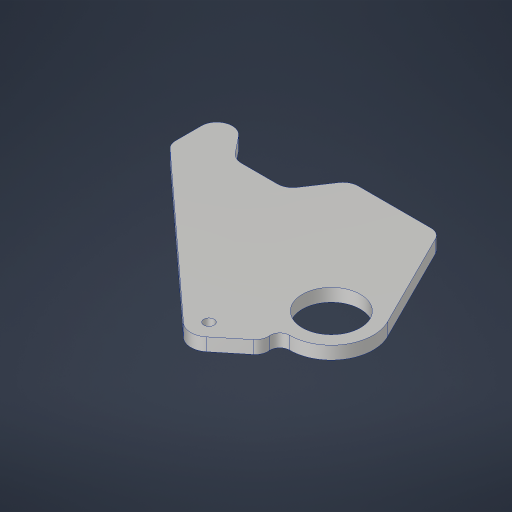
# Autodesk Inventor part: CL4-004
Saved by Autodesk Inventor 2023.4 (Build 274418000, 418)
## iProperties
Created: 2025-02-03
Part Number: CL4-004
Material: Aluminum 6061
Document SubType Name: Modeling
Designer: brand
Density: 2.7 g/cm^3
Appearance: Aluminum - Flat
Author: brand
Autodesk Inventor part; units mm, degrees
ref_plane "YZ Plane" through (0, 0, 0) normal (1, 0, 0) x (0, 1, 0)
ref_plane "XZ Plane" through (0, 0, 0) normal (0, 1, 0) x (-1, 0, 0)
ref_plane "XY Plane" through (0, 0, 0) normal (0, 0, 1) x (1, 0, 0)
sketch "Sketch1" plane through (0, 0, 0) normal (0, 1, 0) x (-1, 0, 0)
  circle A0 centre (76.2, -63.1164) radius 16.7005 construction
  line L0 (63.5, -40.9794) -> (88.9, -40.9794)
  line L1 (88.9, -40.9794) -> (101.6, -56.8544)
  line L2 (101.6, -56.8544) -> (111.125, -56.8544)
  line L3 (111.125, -56.8544) -> (111.125, -31.4544)
  line L4 (111.125, -31.4544) -> (31.4102, 41.4928)
  line L5 (63.5, -40.9794) -> (50.8, -60.0294)
  line L6 (50.8, -60.0294) -> (6.9413, -60.0294)
  circle A1 centre (0, 0) radius 14.2875
  circle A2 centre (0, 0) radius 20.6375 construction
  line L7 (6.9413, -60.0294) -> (-18.4587, -9.2294)
  circle A3 centre (0, 25.4) radius 4.7625 construction
  circle A4 centre (25.4, 34.925) radius 2.5527 construction
  circle A5 centre (25.4, 34.925) radius 8.9027 construction
  line L8 (19.7688, 41.8204) -> (3.5498, 28.575)
  arc A6 (0, 20.6375) -> (3.5498, 28.575) centre (0, 25.4) ccw
  arc A7 (0, 20.6375) -> (-18.4587, -9.2294) centre (0, 0) ccw
  arc A8 (31.4102, 41.4928) -> (19.7688, 41.8204) centre (25.4, 34.925) ccw
  point P0 (76.2, -40.9794)
  dimension "d0" = 33.401
  dimension "d1" = 28.575
  dimension "d2" = 6.35
  dimension "d3" = 9.525
  dimension "d4" = 25.4
  dimension "d5" = 5.1054
  dimension "d6" = 6.35
  dimension "d7" = 25.4
  dimension "d8" = 9.525
  dimension "d9" = 25.4
  dimension "d10" = 50.8
  dimension "d11" = 19.05
  dimension "d12" = 12.7
  dimension "d13" = 25.4
  dimension "d15" = 76.2
  dimension "d16" = 76.2
  dimension "d17" = 12.7
  dimension "d18" = 3.175
  dimension "d19" = 9.525
  dimension "d20" = 25.4
  dimension "d21" = 3.175
  dimension "d22" = 63.1164
  constraints: 18 end point, 10 point on circle, 8 centre point, 4 coincident, 2 horizontal, 2 tangent, 1 concentric, 1 midpoint, 1 parallel, 1 vertical, 1 vertical alignment, 4 other
  measures "d0" diameter of A0
  measures "d1" diameter of A1
  measures "d3" diameter of A3
  measures "d4" distance of A3.centre point (0, 0)
  measures "d5" diameter of A4
  measures "d6" radial gap between concentric circles of A4 A5
  measures "d7" horizontal distance of A4.centre A3.centre
  measures "d8" vertical distance of A3.centre A4.centre
  measures "d9" horizontal distance of L7.end L6.end
  measures "d10" vertical distance of L7.end L6.end
  measures "d11" vertical distance of L0.start L5.end
  measures "d12" horizontal distance of L0.start L5.end
  measures "d13" distance of L0.start L0.end
  measures "d15" horizontal distance of point (0, 0) point (76.2, -40.979)
  measures "d16" horizontal distance of point (0, 0) A0.centre
  measures "d17" horizontal distance of L0.end L1.end
  measures "d18" distance between parallel lines of L6 L2
  measures "d19" distance of L1.end L2.end
  measures "d20" distance of L2.end L3.end
  measures "d21" vertical distance of A3.centre L8.end
  measures "d22" vertical distance of point (0, 0) A0.centre
extrude "Extrusion1" add sketch "Sketch1" against normal blind 6.35
fillet "Fillet1" radius 6.35 4 edges at (-3.5498, -3.175, 28.575) (-6.9413, -3.175, -60.0294) (-111.125, -3.175, -31.4544) (-111.125, -3.175, -56.8544)
fillet "Fillet2" radius 7.62 4 edges at (-63.5, -3.175, -40.9794) (-88.9, -3.175, -40.9794) (-50.8, -3.175, -60.0294) (-101.6, -3.175, -56.8544)
hole "Hole1" at (-25.4, 0, 34.925) direction (0, -1, 0) diameter 5.1054 end through all clearance for "Flat Head Machine Screw (82)" size "#10" standard "Ansi Unified Screw Threads"
equation "\"d17\" = d12"
body "Solid1"
